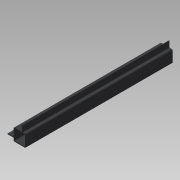
# Autodesk Inventor part: 9010
Saved by Autodesk Inventor 2013 (Build 170138000, 138)
## iProperties
Company: 80/20 Inc.
Created: 2014-04-23
Part Number: 9010
Material: Generic
Document SubType Name: Modeling
Density: 1 g/cm^3
Vendor: 80/20 Inc.
Engineer: Ross Bowman
Designer: Ross Bowman
Catalog Web Link: 8020.net
Material: 6105-T5 Aluminum
Author: Ross Bowman
Keywords: 80/20 , 8020 , T-Slot , Extrusion
Autodesk Inventor part; units mm, degrees
ref_plane "YZ Plane" through (0, 0, 0) normal (1, 0, 0) x (0, 1, 0)
ref_plane "XZ Plane" through (0, 0, 0) normal (0, 1, 0) x (-1, 0, 0)
ref_plane "XY Plane" through (0, 0, 0) normal (0, 0, 1) x (1, 0, 0)
sketch "Sketch1" plane through (0, 0, 0) normal (0, 0, 1) x (1, 0, 0)
  line L0 (11.176, -9.652) -> (11.176, 9.652)
  arc A0 (9.652, -11.176) -> (11.176, -9.652) centre (9.652, -9.652) ccw
  line L1 (-9.652, -11.176) -> (9.652, -11.176)
  arc A1 (-11.176, -9.652) -> (-9.652, -11.176) centre (-9.652, -9.652) ccw
  line L2 (-11.176, 9.652) -> (-11.176, -9.652)
  arc A2 (-9.652, 11.176) -> (-11.176, 9.652) centre (-9.652, 9.652) ccw
  line L3 (9.652, 11.176) -> (-9.652, 11.176)
  arc A3 (11.176, 9.652) -> (9.652, 11.176) centre (9.652, 9.652) ccw
  arc A4 (6.35, 13.462) -> (7.112, 12.7) centre (7.112, 13.462) ccw
  line L4 (6.35, 13.462) -> (6.35, 24.638)
  arc A5 (6.35, 24.638) -> (4.826, 24.638) centre (5.588, 24.638) ccw
  line L5 (4.826, 24.638) -> (4.826, 13.462)
  arc A6 (4.064, 12.7) -> (4.826, 13.462) centre (4.064, 13.462) ccw
  line L6 (4.064, 12.7) -> (-10.5918, 12.7)
  arc A7 (-10.5918, 12.7) -> (-12.7, 10.5918) centre (-10.5918, 10.5918) ccw
  line L7 (-12.7, 10.5918) -> (-12.7, -4.064)
  arc A8 (-13.462, -4.826) -> (-12.7, -4.064) centre (-13.462, -4.064) ccw
  line L8 (-13.462, -4.826) -> (-24.638, -4.826)
  arc A9 (-24.638, -4.826) -> (-24.638, -6.35) centre (-24.638, -5.588) ccw
  line L9 (-24.638, -6.35) -> (-13.462, -6.35)
  arc A10 (-12.7, -7.112) -> (-13.462, -6.35) centre (-13.462, -7.112) ccw
  line L10 (-12.7, -7.112) -> (-12.7, -10.5918)
  arc A11 (-12.7, -10.5918) -> (-10.5918, -12.7) centre (-10.5918, -10.5918) ccw
  line L11 (-10.5918, -12.7) -> (10.5918, -12.7)
  arc A12 (10.5918, -12.7) -> (12.7, -10.5918) centre (10.5918, -10.5918) ccw
  line L12 (12.7, -10.5918) -> (12.7, 10.5918)
  arc A13 (12.7, 10.5918) -> (10.5918, 12.7) centre (10.5918, 10.5918) ccw
  line L13 (10.5918, 12.7) -> (7.112, 12.7)
  point P0 (0, 0)
  constraints: 28 end point, 28 point on circle, 28 tangent, 14 centre point, 10 parallel, 2 collinear, 1 horizontal, 1 vertical
extrude "Extrusion1" add sketch "Sketch1" against normal blind 304.8
body "Solid1"
